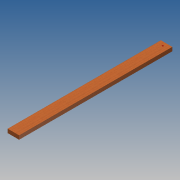
# Autodesk Inventor part: 2p2ps37
Saved by Autodesk Inventor 2014 SP1 (Build 180222100, 222)
## iProperties
Company: HERA Project
Created: 2013-09-03
Part Number: 2p2ps37
Material: Wood (Cherry)
Document SubType Name: Modeling
Designer: Dave
Mass: 2674.39 g
Surface Area: 4094.57 cm^2
Volume: 5348.78 cm^3
Density: 0.5 g/cm^3
Description: Pole stand support 37 degree
Appearance: Cherry - Natural Low Gloss
Author: David DeBoer
Autodesk Inventor part; units mm, degrees
ref_plane "YZ Plane" through (0, 0, 0) normal (1, 0, 0) x (0, 1, 0)
ref_plane "XZ Plane" through (0, 0, 0) normal (0, 1, 0) x (-1, 0, 0)
ref_plane "XY Plane" through (0, 0, 0) normal (0, 0, 1) x (1, 0, 0)
sketch "Sketch1" plane through (0, 0, 0) normal (0, 0, 1) x (1, 0, 0)
  line L0 (0, 0) -> (114, 0)
  line L1 (114, 0) -> (114, 38)
  line L2 (114, 38) -> (0, 38)
  line L3 (0, 38) -> (0, 0)
  dimension "d0" = 114
  dimension "d1" = 38
  constraints: 8 end point, 2 parallel, 1 horizontal, 1 perpendicular
  measures "d0" distance of L0.start L0.end
  measures "d1" distance of L2.end L0.start
extrude "Extrusion1" add sketch "Sketch1" along normal blind 1524
sketch "Sketch3" plane through (0, 38, 0) normal (0, 1, 0) x (1, 0, 0)
  circle A0 centre (57, -38) radius 7.5
  line L0 (114, 0) -> (0, 0) projected
  dimension "d23" = 38
  dimension "d24" = 15
  constraints: 1 centre point
  measures "d23" distance from line of A0.centre L0
  measures "d24" diameter of A0
extrude "Extrusion2" cut sketch "Sketch3" against normal blind 1
body "Solid1"
